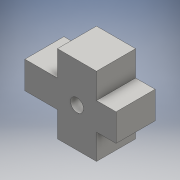
# Autodesk Inventor part: derived_shuttle_6mm
Saved by Autodesk Inventor 2016 (Build 200138000, 138)
## iProperties
Created: 2016-08-02
Part Number: derived_shuttle_6mm
Material: Generic
Document SubType Name: Modeling
Designer: GentnerLab
Density: 1 g/cm^3
Appearance: Default
Author: GentnerLab
Autodesk Inventor part; units mm, degrees
ref_plane "YZ Plane" through (0, 0, 0) normal (1, 0, 0) x (0, 1, 0)
ref_plane "XZ Plane" through (0, 0, 0) normal (0, 1, 0) x (-1, 0, 0)
ref_plane "XY Plane" through (0, 0, 0) normal (0, 0, 1) x (1, 0, 0)
sketch "base+body" plane through (0, 0, 0) normal (0, 1, 0) x (-1, 0, 0)
  circle A0 centre (0, 0) radius 2
  line L0 (-0.75, 1.5) -> (0.75, 1.5)
  line L1 (0.75, 1.5) -> (0.75, -1.5)
  line L2 (0.75, -1.5) -> (-0.75, -1.5)
  line L3 (-0.75, -1.5) -> (-0.75, 1.5)
  line L4 (-0.75, 1.5) -> (0.75, -1.5) construction
  line L5 (0.75, 1.5) -> (-0.75, -1.5) construction
  line L6 (-1.5, 0.525) -> (1.5, 0.525)
  line L7 (1.5, 0.525) -> (1.5, -0.525)
  line L8 (1.5, -0.525) -> (-1.5, -0.525)
  line L9 (-1.5, -0.525) -> (-1.5, 0.525)
  line L10 (-1.5, 0.525) -> (1.5, -0.525) construction
  line L11 (1.5, 0.525) -> (-1.5, -0.525) construction
  line L12 (0, 0.525) -> (2, 0.525)
  line L13 (2, 0.525) -> (2, -0.525)
  line L14 (2, -0.525) -> (0, -0.525)
  line L15 (0, -0.525) -> (0, 0.525)
extrude "Extrusion1" add sketch "base+body" along normal blind 1.5 contours A0 L14 L7 L12 | L13 L14 A0 | A0 L12 L13 | L7 L8 L1 L6 | L6 L3 L0 L1 | L1 L8 L15 L6 | L1 L2 L3 L8 | L15 L8 L3 L6 | L3 L8 L9 L6
derived "zero_sketch.ipt"
sketch "base+body_1" plane through (0, 0, 0) normal (0, 1, 0) x (-1, 0, 0)
  circle A0 centre (0, 0) radius 2 projected
  line L0 (-0.75, 1.5) -> (0.75, 1.5) projected
  line L1 (0.75, 1.5) -> (0.75, -1.5) projected
  line L2 (0.75, -1.5) -> (-0.75, -1.5) projected
  line L3 (-0.75, -1.5) -> (-0.75, 1.5) projected
  line L4 (-0.75, 1.5) -> (0.75, -1.5) construction
  line L5 (0.75, 1.5) -> (-0.75, -1.5) construction
  line L6 (-1.5, 0.525) -> (1.5, 0.525) projected
  line L7 (1.5, 0.525) -> (1.5, -0.525) projected
  line L8 (1.5, -0.525) -> (-1.5, -0.525) projected
  line L9 (-1.5, -0.525) -> (-1.5, 0.525) projected
  line L10 (-1.5, 0.525) -> (1.5, -0.525) construction
  line L11 (1.5, 0.525) -> (-1.5, -0.525) construction
  line L12 (0, 0.525) -> (2, 0.525) projected
  line L13 (2, 0.525) -> (2, -0.525) projected
  line L14 (2, -0.525) -> (0, -0.525) projected
  line L15 (0, -0.525) -> (0, 0.525) projected
hole "Hole1" at (0, 0, 0) direction (0, 1, 0) diameter 0.5 end through all
body "Solid1"
